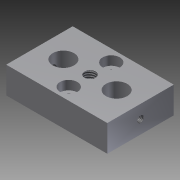
# Autodesk Inventor part: 1_0204_007
Saved by Autodesk Inventor 2012 SP1 (Build 160190100, 190)
## iProperties
Created: 2013-03-27
Part Number: 1_0204_007
Material: Default
Document SubType Name: Modeling
Designer: vogel
Density: 1 g/cm^3
Author: vogel
Autodesk Inventor part; units mm, degrees
ref_plane "YZ Plane" through (0, 0, 0) normal (1, 0, 0) x (0, 1, 0)
ref_plane "XZ Plane" through (0, 0, 0) normal (0, 1, 0) x (-1, 0, 0)
ref_plane "XY Plane" through (0, 0, 0) normal (0, 0, 1) x (1, 0, 0)
sketch "Skizze1" plane through (0, 0, 0) normal (0, 0, 1) x (1, 0, 0)
  line L0 (-19, 12.5) -> (19, 12.5)
  line L1 (19, 12.5) -> (19, -12.5)
  line L2 (19, -12.5) -> (-19, -12.5)
  line L3 (-19, -12.5) -> (-19, 12.5)
  line L4 (-26.6, 0) -> (26.6, 0) projected
  line L5 (0, -17.5) -> (0, 17.5) projected
  point P0 (0, 0)
  dimension "d0" = 25
  dimension "d1" = 38
  constraints: 8 end point, 2 parallel, 1 horizontal, 1 perpendicular, 2 other
  measures "d0" distance of L2.end L0.start
  measures "d1" distance of L1.end L2.end
extrude "Extrusion1" add sketch "Skizze1" along normal blind 10
sketch "Skizze2" plane through (0, 0, 10) normal (0, 0, 1) x (1, 0, 0)
  line L0 (-26.6, 0) -> (26.6, 0) projected
  line L1 (0, -17.5) -> (0, 17.5) projected
  point P0 (0, 0)
  point P1 (-10, 0)
  point P2 (10, 0)
  dimension "d4" = 20
  constraints: 2 point on line, 1 symmetric about line
  measures "d4" distance of point (10, 0) point (-10, 0)
hole "Bohrung1" at (-10, 0, 10) at (10, 0, 10) direction (0, 0, -1) diameter 8 end through all
sketch "Skizze3" plane through (0, 0, 10) normal (0, 0, 1) x (1, 0, 0)
  line L0 (0, -17.5) -> (0, 17.5) projected
  line L1 (-26.6, 0) -> (26.6, 0) projected
  point P0 (0, 0)
  point P1 (0, 8)
  point P2 (0, -8)
  dimension "d28" = 6
  dimension "d12" = 16
  constraints: 2 point on line, 1 symmetric about line
  measures "d12" distance of point (0, -8) point (0, 8)
hole "Bohrung2" at (0, 8, 10) at (0, -8, 10) direction (0, 0, -1) diameter 3.4 end through all counterbore diameter 6.5 counterbore depth 3.4
sketch "Skizze4" plane through (0, 0, 10) normal (0, 0, 1) x (1, 0, 0)
  point P0 (0, 0)
  point P1 (0, 0)
  constraints: 1 coincident
hole "Bohrung3" at (0, 0, 10) direction (0, 0, -1) diameter 4.134 end through all thread size "M5x0.8" class "6H" standard "ISO Metric profile"
sketch "Skizze5" plane through (19, -12.5, 0) normal (1, 0, 0) x (0, 0, -1)
  line L0 (-10, 25) -> (-10, 0) projected
  line L1 (0, 0) -> (-10, 0) projected
  line L2 (0, 25) -> (-10, 25) projected
  line L3 (-10, 12.5) -> (0, 12.5)
  line L4 (-5, 25) -> (-5, 0)
  point P0 (-5, 12.5)
  constraints: 4 end point, 4 midpoint, 1 parallel
hole "Bohrung4" at (19, 0, 5) direction (-1, 0, 0) diameter 2.459 end up to surface thread size "M3x0.5" class "6H" standard "ISO Metric profile"
mirror "Spiegeln2" about plane through (0, 0, 0) normal (1, 0, 0) of "Bohrung4"
